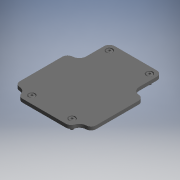
# Autodesk Inventor part: SLZ_63_Abdeckung#
Saved by Autodesk Inventor 2017.3 (Build 213256000, 256)
## iProperties
Part Number: SLZ_63_Abdeckung#
Material: Generic
Catalog Web Link: www.cadenas.de
Description: Abdeckung_SLZ63-Control-Tec
Vendor: ROSEKRIEGER
Document SubType Name: Modeling
Designer: partserver
Manufacturer: ROSEKRIEGER
Mass: 68.1613 g
Surface Area: 310.969 cm^2
Volume: 68.1613 cm^3
Density: 1 g/cm^3
Appearance: PSOLRGB-128-128-128
Category: PARTsolutions
Company: ROSEKRIEGER
Title: SLZ_63_Abdeckung#
Author: Cadenas PARTsolutions
Comments: Control-Tec
PSOL_IDENT_0: {$CADENAS_DATA\23d-libs\rose_krieger\linearkomponenten\pool_lineartechnik\_hubsaeule_zyliinder\elekt
PSOL_IDENT_1: rozylinder\elekzyl_slz63\parts\slz63_plfl_antrieb_abdeckung.prj},183 {VTYP=3D},{NB=SLZ_63_Abdeckung#
PSOL_IDENT_2: },{LINA=SLZ_63_Abdeckung#},{NN=Abdeckung_SLZ63},{DATE=02.12.2020 11:16:22},{GEOMDATE=22.06.2016 13:2
PSOL_IDENT_3: 1:45},{VERSION=},{LINEID=10},{WBVAR=},{WBNUMERIC=}  {NB=SLZ_63_Abdeckung#},{LINA=SLZ_63_Abdeckung#},
PSOL_IDENT_4: {KT=DUMMY},{IDNR=},{CODE=TQ3},{ARTIKEL=Elektrozylinder },{TYPE=SLZ 63 KG P PL},{BEST=SLZ_63_Abdeckun
PSOL_IDENT_5: g},{VARIANTE=PL},{SPINDEL=KG 25x10},{SPINDELCODE=3.000},{SCHUTZARTVIS=IP54},{SCHUTZART=1},{HUB1=0,[0
PSOL_IDENT_6: :100]},{HINWEINBAUX=Hub + 288,5 mm},{DUMMYDURCH=10.000},{DUMMYLAENG=20.000},{HILFEHUB=105},{LAENDOPP
PSOL_IDENT_7: ROFIL=184.500},{RF=1.000},{GRUNDKOE=288.500},{A=100},{B=80},{C=100},{D=125},{E=238},{F=40},{G=M16x1.
PSOL_IDENT_8: 5},{H=104},{K=125},{L=105},{M=48},{N=56.5},{O=86},{P=18.5},{PPATH=sbl_lz70p_plfl.prj}
NB: SLZ_63_Abdeckung#
NN: Abdeckung_SLZ63
NT: Control-Tec
NBSYN: $BEST.#
LINA: SLZ_63_Abdeckung#
CATALOG: RK Rose+Krieger
ARTIKEL: Elektrozylinder
TYPE: SLZ 63 KG P PL
BEST: SLZ_63_Abdeckung
SPINDEL: KG 25x10
SPINDELCODE: 3
SCHUTZARTVIS: IP54
SCHUTZART: 1
HUB1: 0,[0:100]
HINWEINBAUX: Hub + 288,5 mm
DUMMYDURCH: 10
DUMMYLAENG: 20
HILFEHUB: 105
LAENDOPPROFIL: 184.5
RF: 1
GRUNDKOE: 288.5
A: 100
B: 80
C: 100
D: 125
E: 238
F: 40
G: M16x1.5
H: 104
K: 125
L: 105
M: 48
N: 56.5
O: 86
P: 18.5
SUPPLIER: ROSEKRIEGER
ARTICLENO: SLZ_63_Abdeckung#
BOMINFO: SLZ_63_Abdeckung#
CREATOR: CADENAS GmbH
Autodesk Inventor part; units mm, degrees
sketch "Sketch_2" plane through (0, 0, 0) normal (0, 0, 1) x (1, 0, 0)
  line L0 (-57, -93.473) -> (-57, -157.0069)
  arc A0 (-57, -157.0069) -> (-49.7083, -164.5041) centre (-49.5, -157.0069) ccw
  arc A1 (-39.9748, -171.8784) -> (-49.7083, -164.5041) centre (-50, -175) ccw
  arc A2 (-39.9748, -171.8784) -> (-32.3365, -177.5) centre (-32.3365, -169.5) ccw
  line L1 (-32.3365, -177.5) -> (32.3365, -177.5)
  arc A3 (32.3365, -177.5) -> (39.9748, -171.8784) centre (32.3365, -169.5) ccw
  arc A4 (49.7083, -164.5041) -> (39.9748, -171.8784) centre (50, -175) ccw
  arc A5 (49.7083, -164.5041) -> (57, -157.0069) centre (49.5, -157.0069) ccw
  line L2 (57, -157.0069) -> (57, -93.473)
  arc A6 (57, -93.473) -> (49.4324, -85.4846) centre (49, -93.473) ccw
  arc A7 (39.5, -75) -> (49.4324, -85.4846) centre (50, -75) ccw
  line L3 (39.5, -75) -> (39.5, -48.5)
  arc A8 (39.5, -48.5) -> (31.5, -40.5) centre (31.5, -48.5) ccw
  line L4 (31.5, -40.5) -> (-31.5, -40.5)
  arc A9 (-31.5, -40.5) -> (-39.5, -48.5) centre (-31.5, -48.5) ccw
  line L5 (-39.5, -48.5) -> (-39.5, -75)
  arc A10 (-49.4324, -85.4846) -> (-39.5, -75) centre (-50, -75) ccw
  arc A11 (-49.4324, -85.4846) -> (-57, -93.473) centre (-49, -93.473) ccw
  constraints: 24 point on circle, 12 centre point, 12 end point
extrude "Extrusion1" add sketch "Sketch_2" along normal blind 5
sketch "Sketch2" plane through (0, 0, 0) normal (0, 0, -1) x (-1, 0, 0)
  point P0 (-30, -50.2)
hole "Hole1" at (30, -50.2, 0) direction (0, 0, 1) diameter 5.5 depth 5 counterbore diameter 10 counterbore depth 3.5
pattern_linear "Rectangular Pattern1" count 2 spacing 60 along (-1, 0, 0) count 2 spacing 115.8 along (0, -1, 0) of "Hole1"
sketch "Sketch_18" plane through (30, 0, 0) normal (1, 0, 0) x (0, 0, -1)
  line L0 (0, -50.2) -> (-13.5, -50.2)
  line L1 (-13.5, -50.2) -> (-13.5, -48.1905)
  line L2 (-13.5, -48.1905) -> (-13.0095, -47.7)
  line L3 (-13.0095, -47.7) -> (-3.7, -47.7)
  arc A0 (-3.7, -47.7) -> (-3.5, -47.5) centre (-3.7, -47.5) ccw
  line L4 (-3.5, -47.5) -> (-3.5, -46.15)
  arc A1 (-3.3, -45.95) -> (-3.5, -46.15) centre (-3.3, -46.15) ccw
  line L5 (-3.3, -45.95) -> (-0.5, -45.95)
  line L6 (-0.5, -45.95) -> (0, -46.45)
  line L7 (0, -46.45) -> (0, -50.2)
  line L8 (0, -50.2) -> (-13.5, -50.2)
  constraints: 18 end point, 4 point on circle, 2 centre point
revolve "Revolution1" add sketch "Sketch_18" angle 360 about axis through (30, -50.2, 0) along (0, 0, -1)
thread "Thread1" size "M5x0.8" class "6g" standard "ISO Metric profile" length 8.66
pattern_linear "Rectangular Pattern2" count 2 spacing 60 along (-1, 0, 0) count 2 spacing 115.8 along (0, -1, 0) of "Revolution1"
sketch "Sketch_22" plane through (0, 0, 0) normal (0, 0, 1) x (1, 0, 0)
  line L0 (28.5, -51.066) -> (30, -51.9321)
  line L1 (30, -51.9321) -> (31.5, -51.066)
  line L2 (31.5, -51.066) -> (31.5, -49.334)
  line L3 (31.5, -49.334) -> (30, -48.4679)
  line L4 (30, -48.4679) -> (28.5, -49.334)
  line L5 (28.5, -49.334) -> (28.5, -51.066)
  constraints: 12 end point
extrude "Extrusion2" cut sketch "Sketch_22" along normal blind 2.7
pattern_linear "Rectangular Pattern3" count 2 spacing 60 along (-1, 0, 0) count 2 spacing 115.8 along (0, -1, 0) of "Extrusion2"
ref_plane "ANTRIEBABDECKUNG_XY" through (0, 0, 0) normal (0, 0, -1) x (1, 0, 0)
ref_plane "ANTRIEBABDECKUNG_YZ" through (0, 0, 0) normal (1, 0, 0) x (0, -1, 0)
ref_plane "ANTRIEBABDECKUNG_ZX" through (0, 0, 0) normal (0, -1, 0) x (0, 0, -1)
body "Solid1"
